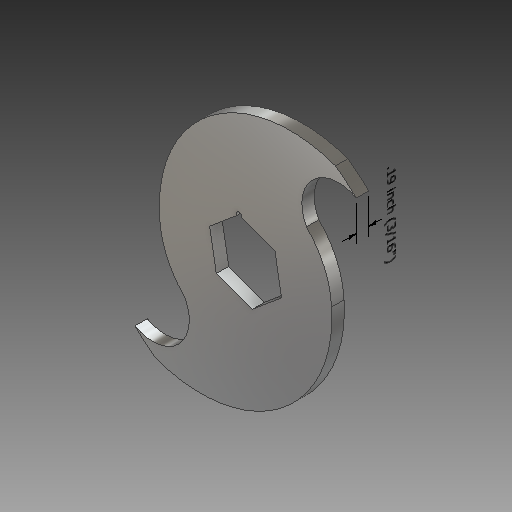
# Autodesk Inventor part: 3-16inch_Knife1_Piece1
Saved by Autodesk Inventor 2018 (Build 220112000, 112)
## iProperties
Created: 2018-01-21
Part Number: 3-16inch_Knife1_Piece1
Material: Generic
Document SubType Name: Modeling
Designer: Olivier
Density: 1 g/cm^3
Appearance: Default
Mass: 22.6609 g
Surface Area: 115.766 cm^2
Volume: 22.6609 cm^3
Author: Olivier
Autodesk Inventor part; units mm, degrees
ref_plane "YZ Plane" through (0, 0, 0) normal (1, 0, 0) x (0, 1, 0)
ref_plane "XZ Plane" through (0, 0, 0) normal (0, 1, 0) x (-1, 0, 0)
ref_plane "XY Plane" through (0, 0, 0) normal (0, 0, 1) x (1, 0, 0)
sketch "Sketch1" plane through (0, 0, 0) normal (0, 0, 1) x (1, 0, 0)
  arc A0 (-32.5736, 42.4264) -> (-51.6655, 23.3345) centre (-39.3901, 30.151) ccw
  arc A1 (-32.5736, 42.4264) -> (-40.5736, 49.1408) centre (-75, 0) ccw
  arc A2 (-40.5736, 49.1408) -> (-107.9651, -1.5164) centre (-57.8736, 2.0002) ccw
  arc A3 (-107.9651, -1.5164) -> (-98.3345, -23.3345) centre (-75, 0) ccw
  arc A4 (-117.4264, -42.4264) -> (-98.3345, -23.3345) centre (-110.6099, -30.151) ccw
  arc A5 (-117.4264, -42.4264) -> (-109.4264, -49.1408) centre (-75, 0) ccw
  arc A6 (-109.4264, -49.1408) -> (-42.0348, 1.5164) centre (-92.1264, -2.0002) ccw
  arc A7 (-42.0348, 1.5164) -> (-51.6655, 23.3345) centre (-75, 0) ccw
  line L0 (-76.6068, 14.0999) -> (-63.7662, 9.4263)
  line L1 (-63.7662, 9.4263) -> (-61.2197, -5.0156)
  line L2 (-61.2197, -5.0156) -> (-72.4535, -14.4419)
  line L3 (-72.4535, -14.4419) -> (-86.2338, -9.4263)
  line L4 (-86.2338, -9.4263) -> (-88.7803, 5.0156)
  line L5 (-88.7803, 5.0156) -> (-78.3125, 13.7991)
  arc A8 (-76.6068, 14.0999) -> (-78.3125, 13.7991) centre (-77.5465, 14.4419) ccw
  arc A9 (-40.5736, 49.1408) -> (-107.9651, -1.5164) centre (-57.8736, 2.0002) ccw
  arc A10 (-107.9651, -1.5164) -> (-98.3345, -23.3345) centre (-75, 0) ccw
  arc A11 (-117.4264, -42.4264) -> (-98.3345, -23.3345) centre (-110.6099, -30.151) ccw
  arc A12 (-117.4264, -42.4264) -> (-109.4264, -49.1408) centre (-75, 0) ccw
  arc A13 (-109.4264, -49.1408) -> (-42.0348, 1.5164) centre (-92.1264, -2.0002) ccw
  arc A14 (-42.0348, 1.5164) -> (-51.6655, 23.3345) centre (-75, 0) ccw
  arc A15 (-32.5736, 42.4264) -> (-51.6655, 23.3345) centre (-39.3901, 30.151) ccw
  arc A16 (-32.5736, 42.4264) -> (-40.5736, 49.1408) centre (-75, 0) ccw
  point P0 (0, 0)
  constraints: 34 point on circle, 17 centre point, 12 end point
extrude "Extrusion1" add sketch "Sketch1" along normal blind 4.7625
body "Solid1"
